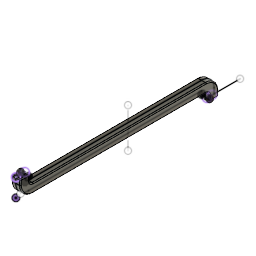
pret_2 (Autodesk Fusion 360 design; units mm, degrees)
part number: 2026-01-05-10-12-13-082
Autodesk Fusion 360 part; units mm, degrees
note: some values were not read from the file. Set by a fixed rule: which sketch regions a step uses.
sketch "Szkic1" plane through (0, 0, 0) normal (1, 0, 0) x (0, 1, 0)
  line L0 (5, 10) -> (0, 10)
  line L1 (0, 10) -> (0, 7)
  line L2 (7, 0) -> (103.5, 0)
  line L3 (110.5, -5) -> (110.5, -2)
  line L4 (103.5, 5) -> (7, 5)
  line L5 (5, 7) -> (5, 10)
  arc A0 (5, 7) -> (7, 5) centre (7, 7) ccw
  arc A1 (0, 7) -> (7, 0) centre (7, 7) ccw
  line L6 (62.5, -8.5) -> (62.5, 13.5) construction
  line L7 (125, -5) -> (105.5, -5)
  line L8 (105.5, -5) -> (105.5, -2)
  arc A2 (110.5, -2) -> (103.5, 5) centre (103.5, -2) ccw
  arc A3 (105.5, -2) -> (103.5, 0) centre (103.5, -2) ccw
  point P0 (5, 5)
  dimension "d2" = 10
  dimension "d24" = 5
  dimension "d25" = 7
  dimension "d26" = 5
  dimension "d33" = 110.5
  dimension "d34" = 62.5
  dimension "d36" = 5
  dimension "d37" = 5
  dimension "d40" = 7
  constraint horizontal L0
  constraint perpendicular L0 L1
  constraint perpendicular L1 L2
  constraint perpendicular L2 L3
  constraint perpendicular L3 L4
  constraint perpendicular L0 L5
  constraint coincident P0 L5
  constraint coincident P0 L4
  constraint tangent L5 A0
  constraint tangent L4 A0
  constraint coincident origin L1
  constraint coincident origin L2
  constraint tangent L1 A1
  constraint tangent L2 A1
  constraint concentric A0 A1
  constraint vertical L6
  constraint perpendicular L2 L8
  constraint horizontal L7
  constraint coincident L3.start L7
  constraint tangent L4 A2
  constraint tangent L3 A2
  constraint tangent L2 A3
  constraint tangent L8 A3
  constraint concentric A2 A3
  measures "d2" distance of L0.end origin
  measures "d24" distance of A0 A1
  measures "d25" radius of A1
  measures "d26" distance of L1 L5
  measures "d33" distance of origin L3
  measures "d34" distance of origin L6
  measures "d36" distance of L2 L7
  measures "d37" distance of L3 L8
  measures "d40" radius of A2
extrude "Wyciągnięcie proste1" add sketch "Szkic1" along normal mid plane 5
sketch "Szkic2" plane through (0, 0, 0) normal (1, 0, 0) x (0, 1, 0)
  line L0 (2.5, 0.7162) -> (2.5, 12.8) construction
  arc A0 (2.5, 9.4) -> (2.5, 12.8) centre (2.5, 11.1) ccw
  line L1 (2.5, 12.8) -> (2.5, 9.4)
  line L2 (5, 10) -> (0, 10)
  dimension "d7" = 3.4
  dimension "d27" = 1.1
  dimension "d28" = 2.5
  constraint vertical L0
  constraint coincident L0 A0.start
  constraint coincident A0.centre L1
  measures "d7" diameter of A0
  measures "d27" distance of A0.centre L2
  measures "d28" horizontal distance of origin A0.centre
revolve "Obrót1" add sketch "Szkic2" angle 360 about axis through (0, 2.5, 0.7162) along (0, 0, 1)
fillet "Zaokrąglenie1" radius 0.5 1 faces at (2.5, 39.1667, 1.6667)
fillet "Zaokrąglenie2" radius 0.5 1 faces at (-2.5, 39.1667, 1.6667)
fillet "Zaokrąglenie3" radius 0.25 1 edges at (-0.4687, 1.2916, 10)
fillet "Zaokrąglenie6" radius 0.5 3 edges at (-2.3536, 4.8536, 9.8536) (0, 5, 10) (2.3536, 4.8536, 9.8536)
fillet "Zaokrąglenie7" radius 0.5 3 edges at (-2.3536, 0.1464, 9.8536) (0, 0, 10) (2.3536, 0.1464, 9.8536)
fillet "Zaokrąglenie8" radius 1 6 edges at (-2.3536, 105.6464, -4.8536) (0, 105.5, -5) (2.3536, 105.6464, -4.8536) (2.3536, 110.3536, -4.8536) (0, 110.5, -5) (-2.3536, 110.3536, -4.8536)
sketch "Szkic3" plane through (0, 0, 0) normal (1, 0, 0) x (0, 1, 0)
  line L0 (108, -4.4) -> (108, -7.8)
  arc A0 (108, -7.8) -> (108, -4.4) centre (108, -6.1) ccw
  line L1 (106.5, -5) -> (109.5, -5)
  circle A1 centre (108, -6.1) radius 1.7 construction
  dimension "d43" = 3.4
  dimension "d44" = 1.1
  dimension "d50" = 1.5
  constraint vertical L0
  constraint coincident A0.centre L0
  constraint concentric A0 A1
  measures "d43" diameter of A0
  measures "d44" distance of A0.centre L1
  measures "d50" distance of L0 L1.start
revolve "Obrót2" add sketch "Szkic3" angle 360 about axis through (0, 108, -4.4) along (0, 0, -1)
fillet "Zaokrąglenie9" radius 0.25 1 edges at (-0.4687, 109.2084, -5)
equation "d34 = ( 125 / 2 ) * 1 mm"
